Autodesk Fusion 360 part; units mm, degrees
(part 2 of 2)
sketch "Skizze18" plane through (0, -1, 0) normal (0, -1, 0) x (1, 0, 0)
  circle A0 centre (0, 0) radius 3.6
  circle A1 centre (0, 0) radius 16.3753
  circle A2 centre (0, 0) radius 16.3753
  circle A3 centre (0, 0) radius 15.8753
  dimension "d117" = 0.5
  measures "d117" distance of A1 A3
extrude "Extrusion19" cut sketch "Skizze18" against normal through all contours A1 A2 bodies 1
sketch "Sketch19" plane through (0, 8, 0) normal (0, 1, 0) x (-1, 0, 0)
  circle A0 centre (0, 0) radius 15.8753
  line L0 (0, 0) -> (0, -9)
  circle A1 centre (0, 0) radius 3.6
  dimension "d125" = 9
  measures "d125" distance of A0.centre
hole "Hole1" at (0, 8, -9) direction (0, -1, 0) diameter 4.2 depth 20 tip angle 118 counterbore diameter 7.2 counterbore depth 4.2 bodies 1
pattern_circular "C-Pattern4" count 4 over 360 about axis through (0, 1.75, 0) along (0, 1, 0) of "Hole1"
equation "d8 = PLD"
equation "teethCount = 33"
equation "PLD = 0.381 mm"
equation "outerDiameter = ( ( pitchLength * teethCount ) / PI ) - ( 2 * PLD )"
equation "pitchLength = 3 mm"
equation "pitchDiameter = ( pitchLength * teethCount ) / PI"
equation "anglePerTooth = 360 deg / teethCount"
equation "d19 = anglePerTooth / 2"
equation "d25 = beltWidth"
equation "d28 = teethCount"
equation "d30 = outerDiameter + 2 mm"
equation "d33 = outerDiameter + 2 mm"
equation "beltWidth = 7 mm"
equation "magicSplintOffset = 10 mm"
equation "magicAxelFactor = 0.5"
equation "holeOffsetToPD = 3 mm"
equation "holeCount = 10"
equation "holeInnerDiameter = 18 mm"
equation "holeToFillRatio = 0.6"
equation "h = 1.14 mm" comment "from datasheet"
equation "i = 1.26 mm" comment "from datasheet"
equation "innerRadius = ( teethCount * pitchLength / PI ) / 2 - h - ( i / 2 )" comment "This expression comes from the lego gt3 wheel design in openscad"
equation "d131 = innerRadius"
named bodies: "GT3_pulley_rev1_gimbal_33T"
